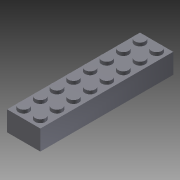
# Autodesk Inventor part: 3007
Saved by Autodesk Inventor 2011 SP1 (Build 150282100, 282)
## iProperties
Company: Allseas Engineering BV
Created: 2011-09-26
Part Number: 3007
Cost Center: 0 kg
Material: Steel
Document SubType Name: Modeling
Designer: PMe
Authority: 0 mm^3
Stock Number: =<Filenr>_<Document number>
Density: 7.85 g/cm^3
Act. Code: DW000
SaveDate: 2011-07-28
SaveTime: 18:32
FileName: Standard
TotalMass: 0 kg
TotalVolume: 0 mm^3
Subject: =<Title><TITLE 1_2> <TITLE 2_2>
Author: PMe
Autodesk Inventor part; units mm, degrees
ref_plane "YZ Plane" through (0, 0, 0) normal (1, 0, 0) x (0, 1, 0)
ref_plane "XZ Plane" through (0, 0, 0) normal (0, 1, 0) x (-1, 0, 0)
ref_plane "XY Plane" through (0, 0, 0) normal (0, 0, 1) x (1, 0, 0)
sketch "Sketch1" plane through (0, 0, 0) normal (0, 0, 1) x (1, 0, 0)
  line L0 (-8, 32) -> (8, 32)
  line L1 (8, 32) -> (8, -32)
  line L2 (8, -32) -> (-8, -32)
  line L3 (-8, -32) -> (-8, 32)
  point P0 (0, 0)
  dimension "d0" = 16
  dimension "d1" = 64
  dimension "d2" = 8
  dimension "d3" = 32
  constraints: 8 end point, 2 parallel, 1 horizontal, 1 perpendicular
  measures "d0" distance of L1.end L2.end
  measures "d1" distance of L0.end L1.end
  measures "d2" distance from line of point (0, 0) L1
  measures "d3" distance from line of point (0, 0) L2
extrude "Extrusion1" add sketch "Sketch1" along normal blind 9.6
shell "Shell1" thickness 1.5 removed faces 1 at (-2.6667, 10.6667, 0)
sketch "Sketch2" plane through (0, 0, 9.6) normal (0, 0, 1) x (1, 0, 0)
  circle A0 centre (4, -28) radius 2.5
  line L0 (8, 32) -> (8, -32) projected
  line L1 (8, -32) -> (-8, -32) projected
  dimension "d7" = 5
  dimension "d10" = 4
  dimension "d11" = 4
  constraints: 1 centre point, 1 coincident
  measures "d7" diameter of A0
  measures "d10" distance from line of L1 point (4, -28)
  measures "d11" distance from line of L0 point (4, -28)
extrude "Extrusion2" add sketch "Sketch2" along normal blind 1.6
sketch "Sketch3" plane through (6.5, -30.5, 8.1) normal (0, 0, -1) x (-1, 0, 0)
  circle A0 centre (2.5, 2.5) radius 2.5 projected
  circle A1 centre (2.5, 2.5) radius 1.2
  point P0 (6.5, 30.5)
  dimension "d18" = 2.4
  constraints: 1 centre point, 1 coincident
  measures "d18" diameter of A1
extrude "Extrusion3" cut sketch "Sketch3" against normal blind 1.6 contours A1
pattern_linear "Rectangular Pattern1" count 8 spacing 8 along (0, 1, 0) count 2 spacing 8 along (-1, 0, 0) of "Extrusion2", "Extrusion3"
sketch "Sketch4" plane through (6.5, -30.5, 8.1) normal (0, 0, -1) x (-1, 0, 0)
  circle A0 centre (2.5, 10.5) radius 1.2 projected
  circle A1 centre (2.5, 2.5) radius 1.2 projected
  line L0 (0, 61) -> (0, 0) projected
  line L1 (0, 0) -> (13, 0) projected
  circle A2 centre (6.5, 6.5) radius 3.15
  circle A3 centre (6.5, 6.5) radius 2.5
  point P0 (6.5, 30.5)
  dimension "d21" = 6.5
  dimension "d22" = 6.5
  dimension "d23" = 10.5
  dimension "d24" = 2.5
  dimension "d25" = 5
  dimension "d26" = 6.3
  constraints: 2 centre point, 1 coincident
  measures "d21" distance from line of L1 A2.centre
  measures "d22" distance from line of L0 A2.centre
  measures "d23" distance from line of L1 A0.centre
  measures "d24" distance from line of L1 A1.centre
  measures "d25" diameter of A3
  measures "d26" diameter of A2
extrude "Extrusion4" add sketch "Sketch4" along normal up to surface (8.1 mm away) contours A2
pattern_linear "Rectangular Pattern2" count 7 spacing 8 along (0, 1, 0) of "Extrusion4"
equation "\"d0\" = 8 * WIDTH"
equation "\"d1\" = 8 * LENGTH"
equation "\"d2\" = 0.5 * d0"
equation "\"d3\" = 0.5 * d1"
equation "\"d21\" = 0.5 * d23 + 0.5 * d24"
equation "\"d22\" = d21"
equation "\"WIDTH\" = 2"
equation "\"LENGTH\" = 8"
body "Solid1"
